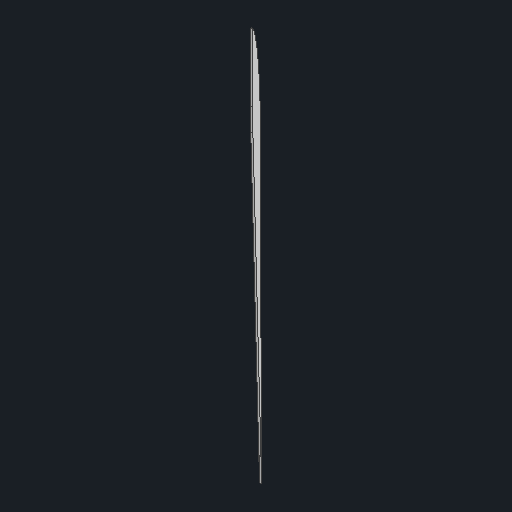
# Autodesk Inventor part: standoff
Saved by Autodesk Inventor 2023 (Build 270158030, 158C)
## iProperties
Created: 2022-03-24
Part Number: standoff
Material: Generic
Document SubType Name: Modeling
Designer: kardo
Density: 1 g/cm^3
Appearance: Default
Author: kardo
Autodesk Inventor part; units mm, degrees
ref_plane "YZ Plane" through (0, 0, 0) normal (1, 0, 0) x (0, 1, 0)
ref_plane "XZ Plane" through (0, 0, 0) normal (0, 1, 0) x (-1, 0, 0)
ref_plane "XY Plane" through (0, 0, 0) normal (0, 0, 1) x (1, 0, 0)
derived "parameters_frame.ipt"
derived "surface_body.ipt"
sketch "sk_rail_bottom_standoff" plane through (34.32, 0, 0) normal (1, 0, 0) x (0, 1, 0)
  line L0 (-363, 18.496) -> (-275.8801, 20.463)
  arc A0 (-275.8801, 20.463) -> (-254.1001, 21.0191) centre (-359.1231, 3707.4463) ccw
  line L1 (30.81, 28.832) -> (94.8, 28.832)
  arc A1 (30.81, 28.832) -> (9.48, 28.5282) centre (30.81, -720.1791) ccw
  line L2 (-254.1001, 21.0191) -> (9.48, 28.5282)
  line L3 (-483, 0) -> (357, 0) construction
  line L4 (9.48, 28.5282) -> (9.48, 0) construction
  line L5 (-254.1001, 21.0191) -> (-254.1001, 0) construction
  point P0 (0, 0)
  point P1 (-254.1001, 20.9547)
  point P2 (9.48, 28.832)
sketch "sk_rail_standoff_standoff" plane through (34.32, 0, 0) normal (1, 0, 0) x (0, 1, 0)
  line L0 (0, 21.4767) -> (77.736, 21.7019) construction
  line L1 (77.736, 21.7019) -> (94.8, 28.832) construction
  line L2 (0, 21.4767) -> (-254.1001, 20.7404)
  line L3 (-275.8801, 20.463) -> (-363, 18.496)
  arc A0 (-254.1001, 20.7404) -> (-275.8801, 20.463) centre (-250.8921, -1086.298) ccw
  line L4 (-483, 0) -> (357, 0) construction
  line L5 (-254.1001, 20.7404) -> (-254.1001, 0) construction
  spline S0 degree 2 poles (0, 21.4767) (77.736, 21.7019) (94.8, 28.832) knots 1 1 1 2 2 2
  point P0 (0, 0)
  point P1 (-254.1001, 20.9547)
ref_plane "plane_standoff_right" through (34.32, 0, 0) normal (1, 0, 0) x (0, 1, 0)
sketch "sk_base" plane through (34.32, 0, 0) normal (1, 0, 0) x (0, 1, 0)
  arc A0 (-254.1001, 20.7404) -> (-275.8801, 20.463) centre (-250.8921, -1086.298) ccw construction
  arc A1 (-275.8801, 20.463) -> (-254.1001, 21.0191) centre (-359.1231, 3707.4463) ccw construction
  line L0 (-254.1001, 21.0191) -> (9.48, 28.5282) construction
  line L1 (0, 21.4767) -> (-254.1001, 20.7404) construction
  spline S0 degree 2 poles (0, 21.4767) (77.736, 21.7019) (94.8, 28.832) knots 1 1 1 2 2 2 construction
  line L2 (30.81, 28.832) -> (94.8, 28.832) construction
  arc A2 (30.81, 28.832) -> (9.48, 28.5282) centre (30.81, -720.1791) ccw construction
  line L3 (-0.0035, 22.6767) -> (-254.1036, 21.9403)
  arc A3 (-254.1036, 21.9403) -> (-275.8801, 21.6633) centre (-250.8921, -1086.298) ccw
  arc A4 (-275.8801, 21.6633) -> (-254.1343, 22.2186) centre (-359.1231, 3707.4463) ccw
  line L4 (-254.1343, 22.2186) -> (9.4458, 29.7277)
  arc A5 (30.81, 30.032) -> (9.4458, 29.7277) centre (30.81, -720.1791) ccw
  line L5 (30.81, 30.032) -> (92.8, 30.032)
  line L6 (-275.8801, 20.463) -> (-275.8801, 21.6633) construction
  line L7 (92.8, 29.3559) -> (92.8, 30.032)
  spline S1 degree 5 poles (92.8, 29.3559) (91.3387, 28.8495) (89.8462, 28.4324) (88.3449, 28.0616) (84.0673, 27.1297) (79.7429, 26.4432) (76.9388, 26.059) (70.3634, 25.2737) (63.7659, 24.6977) (59.9843, 24.415) (51.4508, 23.8655) (42.9082, 23.4795) (38.1523, 23.3032) (27.6692, 22.9857) (17.1827, 22.8021) (11.4541, 22.7339) (5.7254, 22.6933) (-0.0035, 22.6767) knots 0 0 0 0 0 0 0.082904 0.082904 0.082904 0.23458 0.23458 0.23458 0.437833 0.437833 0.437833 0.692922 0.692922 0.692922 1 1 1 1 1 1
  point P0 (0, 0)
  dimension "d5" = 1.2
  dimension "d4" = 1.2
  dimension "d6" = 2
  constraints: 10 end point, 6 point on circle, 3 centre point, 2 vertical, 1 parallel, 7 other
  measures "d4" distance between parallel lines of L0 L4
  measures "d6" distance from line of L7 point (94.8, 28.832)
extrude "thicken" add sketch "sk_base" against normal blind 2
equation "\"d4\" = shell_thickness"
equation "\"d6\" = bulkhead_thickness"
equation "\"d2\" = bulkhead_thickness"
equation "\"shell_thickness\" = 1.2"
equation "\"bulkhead_thickness\" = 2"
body "Solid1"
